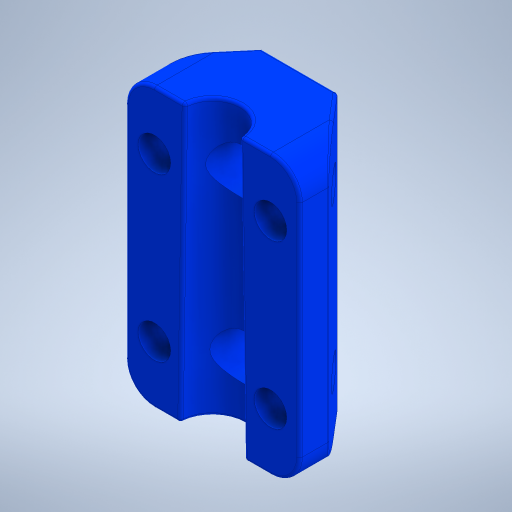
# Autodesk Inventor part: BracketSolderingIron_1
Saved by Autodesk Inventor 2024 (Build 280153000, 153)
## iProperties
Created: 2023-12-27
Part Number: BracketSolderingIron_1
Material: Generisch
Document SubType Name: Modeling
Designer: denni
Density: 1 g/cm^3
Appearance: Vorgabe(1)
Author: denni
Autodesk Inventor part; units mm, degrees
ref_plane "YZ Plane" through (0, 0, 0) normal (1, 0, 0) x (0, 1, 0)
ref_plane "XZ Plane" through (0, 0, 0) normal (0, 1, 0) x (-1, 0, 0)
ref_plane "XY Plane" through (0, 0, 0) normal (0, 0, 1) x (1, 0, 0)
sketch "Skizze1" plane through (0, 0, 0) normal (0, 1, 0) x (-1, 0, 0)
  line L0 (15, 0) -> (-15, 0)
  line L1 (-15, 0) -> (-15, -5)
  line L2 (-15, -5) -> (-6.5, -15)
  line L3 (-6.5, -15) -> (6.5, -15)
  line L4 (6.5, -15) -> (15, -5)
  line L5 (15, -5) -> (15, 0)
  line L6 (0, -15) -> (0, 0) construction
  dimension "d0" = 13
  dimension "d1" = 30
  dimension "d2" = 5
  dimension "d3" = 15
  constraints: 14 end point, 2 equal length, 2 midpoint, 2 parallel, 1 coincident, 1 horizontal, 1 perpendicular
  measures "d0" distance of L2.end L3.end
  measures "d1" distance of L0.start L0.end
  measures "d2" distance of L4.end L0.start
  measures "d3" distance between parallel lines of L0 L3
extrude "Extrusion1" add sketch "Skizze1" along normal blind 48
sketch "Skizze2" plane through (0, 48, 0) normal (0, 1, 0) x (1, 0, 0)
  circle A0 centre (0, 0) radius 4.75
  dimension "d6" = 9.5
  constraints: 1 centre point, 1 coincident
  measures "d6" diameter of A0
sketch "Skizze3" plane through (0, 0, 0) normal (0, -1, 0) x (1, 0, 0)
  circle A0 centre (0, 0) radius 5.5
  dimension "d7" = 11
  constraints: 1 centre point, 1 coincident
  measures "d7" diameter of A0
loft "Erhebung1" cut profiles "Skizze3", "Skizze2"
sketch "Skizze4" plane through (6.5, 0, 0) normal (0, 0, -1) x (-1, 0, 0)
  line L0 (1.75, 48) -> (11.25, 48) construction
  line L1 (6.5, 48) -> (6.5, 38) construction
  line L2 (6.5, 38) -> (6.5, 10) construction
  line L3 (6.5, 10) -> (6.5, 0) construction
  dimension "d21" = 10
  constraints: 6 end point, 2 coincident, 2 collinear, 1 midpoint, 1 perpendicular
  measures "d21" distance from line of L0 point (6.5, 38)
hole "Bohrung1" at (0, 38, 0) at (0, 10, 0) direction (0, 0, -1) diameter 4.5 end through all counterbore diameter 8 counterbore depth 10 clearance for "Inbusschraube ISO 4762" size "M4" standard "ISO"
sketch "Skizze5" plane through (-15, 0, 0) normal (0, 0, 1) x (1, 0, 0)
  line L0 (30, 0) -> (0, 0) construction
  line L1 (0, 0) -> (0, 48) construction
  line L2 (0, 48) -> (30, 48) construction
  line L3 (30, 48) -> (30, 0) construction
  line L4 (30, 0) -> (0, 48) construction
  line L5 (0, 0) -> (30, 48) construction
  line L6 (25, 10) -> (5, 10) construction
  line L7 (5, 10) -> (5, 38) construction
  line L8 (5, 38) -> (25, 38) construction
  line L9 (25, 38) -> (25, 10) construction
  line L10 (25, 10) -> (5, 38) construction
  line L11 (5, 10) -> (25, 38) construction
  point P0 (15, 0)
  point P1 (15, 24)
  point P2 (15, 24)
  dimension "d22" = 5
  dimension "d23" = 10
  constraints: 24 end point, 6 coincident, 5 midpoint, 4 parallel, 2 horizontal, 2 perpendicular
  measures "d22" distance between parallel lines of L1 L7
  measures "d23" distance between parallel lines of L2 L8
hole "Bohrung2" at (-10, 38, 0) at (10, 38, 0) at (10, 10, 0) at (-10, 10, 0) direction (0, 0, -1) diameter 5.6 depth 5
hole "Bohrung3" at (10, 38, 0) at (-10, 38, 0) at (-10, 10, 0) at (10, 10, 0) direction (0, 0, -1) diameter 4.5 end through all clearance for "Inbusschraube ISO 4762" size "M4" standard "ISO"
fillet "Rundung1" radius 5 4 edges at (-15, 0, -2.5) (15, 0, -2.5) (-15, 48, -2.5) (15, 48, -2.5)
fillet "Rundung2" radius 0.5 27 edges at (0, 48, -4.75) (-5.125, 24, 0) (5.125, 24, 0) (13.5355, 46.5355, 0) (15, 24, 0) (13.5355, 1.4645, 0) (7.75, 0, 0) (7.375, 48, 0) (-7.375, 48, 0) (-15, 24, 0) (-13.5355, 1.4645, 0) (-7.75, 0, 0) (-13.5355, 46.5355, 0) (0, 0, -5.5) (-8.25, 0, -12.9412) (-15, 24, -5) (-13.5355, 46.5355, -6.7229) (-8.25, 48, -12.9412) (-13.5355, 1.4645, -6.7229) (13.5355, 46.5355, -6.7229) (15, 24, -5) (13.5355, 1.4645, -6.7229) (8.25, 0, -12.9412) (8.25, 48, -12.9412) (6.5, 24, -15) (0, 48, -15) (0, 0, -15)
